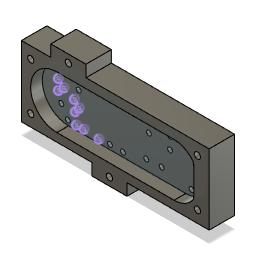
dictofun_1.3_bed_of_nails (Autodesk Fusion 360 design; units mm, degrees)
Autodesk Fusion 360 part; units mm, degrees
(part 1 of 13)
sketch "Sketch1" plane through (0, 0, 0) normal (0, 0, 1) x (1, 0, 0)
  line L0 (139.726, -70.9365) -> (139.721, -70.9397)
  line L1 (139.346, -71.4753) -> (139.289, -71.688)
  line L2 (139.439, -72.5391) -> (139.442, -72.5436)
  line L3 (139.536, -72.6768) -> (139.565, -72.7194)
  line L4 (139.906, -70.811) -> (139.906, -70.811)
  line L5 (139.439, -71.2757) -> (139.437, -71.2807)
  line L6 (139.442, -72.5436) -> (139.442, -72.5436)
  line L7 (139.846, -72.9625) -> (139.89, -73.018)
  line L8 (139.562, -71.0999) -> (139.468, -71.2339)
  line L9 (141.501, -71.0954) -> (141.345, -70.9397)
  line L10 (139.437, -72.5341) -> (139.439, -72.5391)
  line L11 (141.72, -72.3395) -> (141.777, -72.1268)
  line L12 (139.721, -70.9397) -> (139.565, -71.0954)
  line L13 (139.395, -71.3702) -> (139.346, -71.4753)
  line L14 (139.873, -80.9148) -> (139.782, -81.0293)
  line L15 (139.437, -71.2807) -> (139.437, -71.2807)
  line L16 (139.437, -71.2807) -> (139.395, -71.3702)
  line L17 (139.348, -72.3445) -> (139.437, -72.5341)
  line L18 (139.779, -72.9157) -> (139.846, -72.9625)
  line L19 (139.289, -71.688) -> (139.27, -71.9074)
  line L20 (139.565, -71.0954) -> (139.562, -71.0999)
  line L21 (139.78, -81.0344) -> (139.78, -81.0344)
  line L22 (137.742, -83.535) -> (137.082, -82.8744)
  line L23 (136.527, -82.247) -> (136.522, -82.2439)
  line L24 (139.89, -73.018) -> (139.9, -73.0658)
  line L25 (136.966, -82.6541) -> (136.891, -82.5531)
  line L26 (136.848, -82.4955) -> (136.848, -82.4955)
  line L27 (139.9, -73.0658) -> (139.9, -80.8368)
  line L28 (139.565, -72.7194) -> (139.721, -72.8751)
  line L29 (139.687, -81.2096) -> (139.627, -81.4041)
  line L30 (137.057, -82.8364) -> (137.056, -82.8368)
  line L31 (136.628, -82.3102) -> (136.527, -82.247)
  line L32 (137.788, -83.564) -> (137.742, -83.535)
  line L33 (139.437, -72.5341) -> (139.437, -72.5341)
  line L34 (136.522, -82.2439) -> (136.333, -82.1684)
  line L35 (136.969, -82.6593) -> (136.966, -82.6541)
  line L36 (139.748, -81.0945) -> (139.687, -81.2096)
  line L37 (137.056, -82.8368) -> (136.969, -82.6593)
  line L38 (137.921, -83.535) -> (137.858, -83.5691)
  line L39 (137.082, -82.8744) -> (137.057, -82.8364)
  line L40 (139.289, -72.1268) -> (139.346, -72.3395)
  line L41 (139.78, -81.0344) -> (139.748, -81.0945)
  line L42 (139.726, -72.8783) -> (139.726, -72.8783)
  line L43 (139.9, -80.8368) -> (139.88, -80.905)
  line L44 (139.609, -81.6902) -> (139.615, -81.7805)
  line L45 (139.782, -81.0293) -> (139.78, -81.0344)
  line L46 (136.891, -82.5531) -> (136.848, -82.4955)
  line L47 (136.333, -82.1684) -> (136.133, -82.1286)
  line L48 (136.848, -82.4955) -> (136.844, -82.4909)
  line L49 (137.858, -83.5691) -> (137.788, -83.564)
  line L50 (136.844, -82.4909) -> (136.695, -82.3526)
  line L51 (139.627, -81.4041) -> (139.603, -81.6065)
  line L52 (139.599, -81.8497) -> (139.578, -81.8778)
  line L53 (136.105, -81.7081) -> (136.105, -81.7081)
  line L54 (136.128, -82.1286) -> (136.122, -82.128)
  line L55 (136.108, -81.6604) -> (136.11, -81.6482)
  line L56 (136.105, -81.7081) -> (136.107, -81.7004)
  line L57 (139.721, -72.8751) -> (139.726, -72.8783)
  line L58 (139.726, -72.8783) -> (139.779, -72.9157)
  line L59 (139.603, -81.6065) -> (139.609, -81.6902)
  line L60 (139.27, -71.9074) -> (139.289, -72.1268)
  line L61 (139.88, -80.905) -> (139.873, -80.9148)
  line L62 (136.133, -82.1286) -> (136.128, -82.1286)
  line L63 (139.562, -71.0999) -> (139.562, -71.0999)
  line L64 (139.442, -72.5436) -> (139.536, -72.6768)
  line L65 (139.578, -81.8778) -> (137.921, -83.535)
  line L66 (136.527, -82.247) -> (136.527, -82.247)
  line L67 (139.346, -72.3395) -> (139.348, -72.3445)
  line L68 (136.695, -82.3526) -> (136.628, -82.3102)
  line L69 (136.122, -82.128) -> (136.122, -82.1254)
  line L70 (139.468, -71.2339) -> (139.439, -71.2757)
  line L71 (139.615, -81.7805) -> (139.599, -81.8497)
  line L72 (136.127, -72.9976) -> (136.161, -72.9625)
  line L73 (136.046, -81.8942) -> (136.067, -81.8554)
  line L74 (136.065, -82.1077) -> (136.019, -82.0534)
  line L75 (136.083, -81.8058) -> (136.087, -81.7985)
  line L76 (136.023, -81.9456) -> (136.023, -81.9454)
  line L77 (136.088, -81.7907) -> (136.094, -81.7548)
  line L78 (136.096, -81.7432) -> (136.105, -81.7081)
  line L79 (136.088, -81.7907) -> (136.088, -81.7907)
  line L80 (136.069, -81.8477) -> (136.069, -81.8477)
  line L81 (136.161, -72.9625) -> (136.228, -72.9157)
  line L82 (136.112, -81.6404) -> (136.107, -81.5964)
  line L83 (136.564, -72.5436) -> (136.564, -72.5436)
  line L84 (136.087, -81.7985) -> (136.088, -81.7907)
  line L85 (136.01, -81.983) -> (136.023, -81.9456)
  line L86 (136.57, -72.5341) -> (136.658, -72.3445)
  line L87 (136.718, -72.1268) -> (136.737, -71.9074)
  line L88 (136.228, -72.9157) -> (136.281, -72.8783)
  line L89 (136.107, -73.0658) -> (136.127, -72.9976)
  line L90 (136.107, -81.5845) -> (136.107, -73.0658)
  line L91 (136.11, -81.6482) -> (136.112, -81.6404)
  line L92 (136.072, -81.8358) -> (136.079, -81.8171)
  line L93 (136.122, -82.1254) -> (136.065, -82.1077)
  line L94 (136.067, -81.8554) -> (136.069, -81.8477)
  line L95 (136.079, -81.8171) -> (136.083, -81.8058)
  line L96 (136.019, -82.0534) -> (136.01, -81.983)
  line L97 (136.094, -81.7548) -> (136.096, -81.7432)
  line L98 (136.107, -81.7004) -> (136.107, -81.6801)
  line L99 (136.107, -81.6801) -> (136.108, -81.6604)
  line L100 (136.023, -81.9454) -> (136.023, -81.9454)
  line L101 (136.069, -81.8477) -> (136.072, -81.8358)
  line L102 (136.57, -72.5341) -> (136.57, -72.5341)
  line L103 (136.281, -72.8783) -> (136.281, -72.8783)
  line L104 (136.281, -72.8783) -> (136.285, -72.8751)
  line L105 (136.023, -81.9454) -> (136.041, -81.9048)
  line L106 (136.285, -70.9397) -> (136.105, -70.8133)
  line L107 (136.285, -72.8751) -> (136.441, -72.7194)
  line L108 (136.567, -72.5391) -> (136.57, -72.5341)
  line L109 (136.107, -81.5964) -> (136.107, -81.5845)
  line L110 (136.105, -70.8133) -> (135.906, -70.7203)
  line L111 (135.906, -70.7203) -> (135.693, -70.6633)
  line L112 (135.468, -70.6446) -> (135.462, -70.6446)
  line L113 (136.041, -81.9048) -> (136.046, -81.8942)
  line L114 (152.42, -70.6251) -> (152.301, -70.4493)
  line L115 (135.473, -70.6441) -> (135.468, -70.6446)
  line L116 (136.718, -71.688) -> (136.661, -71.4753)
  line L117 (136.471, -72.6768) -> (136.564, -72.5436)
  line L118 (152.642, -69.2633) -> (152.654, -69.3169)
  line L119 (136.661, -72.3395) -> (136.718, -72.1268)
  line L120 (136.441, -72.7194) -> (136.471, -72.6768)
  line L121 (151.93, -70.1136) -> (151.926, -70.1105)
  line L122 (152.129, -70.2665) -> (152.125, -70.2628)
  line L123 (135.462, -70.6446) -> (135.462, -70.6434)
  line L124 (136.564, -72.5436) -> (136.567, -72.5391)
  line L125 (136.444, -71.0999) -> (136.441, -71.0954)
  line L126 (152.442, -70.6493) -> (152.42, -70.6251)
  line L127 (152.301, -70.4493) -> (152.298, -70.4451)
  line L128 (152.506, -70.679) -> (152.442, -70.6493)
  line L129 (152.121, -70.2598) -> (151.93, -70.1136)
  line L130 (135.351, -69.3736) -> (135.405, -69.3271)
  line L131 (152.527, -69.1905) -> (152.595, -69.21)
  line L132 (136.444, -71.0999) -> (136.444, -71.0999)
  line L133 (136.567, -71.2757) -> (136.538, -71.2339)
  line L134 (135.693, -70.6633) -> (135.473, -70.6441)
  line L135 (136.737, -71.9074) -> (136.718, -71.688)
  line L136 (136.661, -71.4753) -> (136.612, -71.3702)
  line L137 (136.538, -71.2339) -> (136.444, -71.0999)
  line L138 (136.57, -71.2807) -> (136.567, -71.2757)
  line L139 (136.612, -71.3702) -> (136.57, -71.2807)
  line L140 (135.331, -69.4417) -> (135.351, -69.3736)
  line L141 (136.441, -71.0954) -> (136.285, -70.9397)
  line L142 (135.456, -69.3157) -> (152.527, -69.1905)
  line L143 (151.7, -69.9904) -> (151.473, -69.912)
  line L144 (136.658, -72.3445) -> (136.661, -72.3395)
  line L145 (152.63, -70.6227) -> (152.576, -70.6691)
  line L146 (135.462, -70.6434) -> (135.399, -70.6306)
  line L147 (136.57, -71.2807) -> (136.57, -71.2807)
  line L148 (135.405, -69.3271) -> (135.456, -69.3157)
  line L149 (152.595, -69.21) -> (152.642, -69.2633)
  line L150 (151.93, -70.1136) -> (151.93, -70.1136)
  line L151 (135.348, -70.5812) -> (135.331, -70.519)
  line L152 (141.63, -71.2807) -> (141.629, -71.2807)
  line L153 (141.504, -71.0999) -> (141.501, -71.0954)
  line L154 (141.668, -81.0591) -> (141.665, -81.0539)
  line L155 (141.805, -81.8497) -> (141.828, -81.6939)
  line L156 (141.225, -80.6462) -> (141.178, -80.5929)
  line L157 (141.811, -81.4327) -> (141.755, -81.2366)
  line L158 (141.777, -72.1268) -> (141.796, -71.9074)
  line L159 (141.629, -71.2807) -> (141.627, -71.2757)
  line L160 (141.72, -71.4753) -> (141.671, -71.3702)
  line L161 (139.901, -70.8133) -> (139.897, -70.8165)
  line L162 (139.897, -70.8165) -> (139.726, -70.9365)
  line L163 (140.533, -70.6441) -> (140.314, -70.6633)
  line L164 (139.897, -70.8165) -> (139.897, -70.8165)
  line L165 (141.718, -72.3445) -> (141.72, -72.3395)
  line L166 (141.627, -71.2757) -> (141.598, -71.2339)
  line L167 (141.598, -71.2339) -> (141.504, -71.0999)
  line L168 (141.345, -70.9397) -> (141.165, -70.8133)
  line L169 (141.187, -72.9976) -> (141.22, -72.9625)
  line L170 (141.63, -72.5341) -> (141.718, -72.3445)
  line L171 (140.965, -70.7203) -> (140.752, -70.6633)
  line L172 (141.167, -80.5396) -> (141.167, -73.0658)
  line L173 (141.884, -81.999) -> (141.827, -81.9564)
  line L174 (141.671, -71.3702) -> (141.63, -71.2807)
  line L175 (141.777, -71.688) -> (141.72, -71.4753)
  line L176 (140.101, -70.7203) -> (140.008, -70.7638)
  line L177 (141.796, -71.9074) -> (141.777, -71.688)
  line L178 (140.314, -70.6633) -> (140.101, -70.7203)
  line L179 (140.752, -70.6633) -> (140.533, -70.6441)
  line L180 (140.008, -70.7638) -> (139.906, -70.811)
  line L181 (139.906, -70.811) -> (139.901, -70.8133)
  line L182 (139.726, -70.9365) -> (139.726, -70.9365)
  line L183 (141.629, -72.5341) -> (141.63, -72.5341)
  line L184 (141.504, -71.0999) -> (141.504, -71.0999)
  line L185 (141.165, -70.8133) -> (140.965, -70.7203)
  line L186 (151.238, -96.6842) -> (151.233, -96.6793)
  line L187 (151.626, -97.4609) -> (151.621, -97.4545)
  line L188 (151.682, -97.5383) -> (151.66, -97.5002)
  line L189 (150.656, -96.4497) -> (150.588, -96.4297)
  line L190 (151.073, -96.5644) -> (150.91, -96.4921)
  line L191 (151.697, -97.5595) -> (151.689, -97.5482)
  line L192 (150.724, -96.4511) -> (150.717, -96.4497)
  line L193 (151.079, -96.5671) -> (151.073, -96.5644)
  line L194 (150.53, -96.3237) -> (150.53, -96.3063)
  line L195 (150.542, -96.376) -> (150.53, -96.3237)
  line L196 (150.838, -95.573) -> (150.818, -95.3831)
  line L197 (150.659, -96.1149) -> (150.664, -96.11)
  line L198 (151.646, -97.4859) -> (151.633, -97.4709)
  line L199 (151.073, -96.5644) -> (151.073, -96.5644)
  line L200 (151.533, -97.3335) -> (151.516, -97.1748)
  line L201 (151.516, -97.1748) -> (151.516, -97.1748)
  line L202 (150.717, -96.4497) -> (150.656, -96.4497)
  line L203 (151.689, -97.5482) -> (151.682, -97.5383)
  line L204 (150.756, -95.9503) -> (150.759, -95.9446)
  line L205 (150.759, -95.9446) -> (150.818, -95.763)
  line L206 (150.818, -95.763) -> (150.824, -95.7052)
  line L207 (151.516, -97.1683) -> (151.457, -96.9866)
  line L208 (150.53, -96.3063) -> (150.551, -96.2382)
  line L209 (151.238, -96.6842) -> (151.238, -96.6842)
  line L210 (151.731, -97.6206) -> (151.722, -97.6028)
  line L211 (151.578, -97.4183) -> (151.569, -97.4094)
  line L212 (151.621, -97.4545) -> (151.587, -97.4263)
  line L213 (151.516, -97.1748) -> (151.516, -97.1683)
  line L214 (151.535, -97.3471) -> (151.533, -97.3335)
  line L215 (151.233, -96.6793) -> (151.079, -96.5671)
  line L216 (151.66, -97.5002) -> (151.646, -97.4859)
  line L217 (151.569, -97.4094) -> (151.535, -97.3471)
  line L218 (151.457, -96.9866) -> (151.361, -96.8213)
  line L219 (150.54, -94.8991) -> (150.54, -94.8991)
  line L220 (150.818, -95.3831) -> (150.759, -95.2015)
  line L221 (150.659, -96.1149) -> (150.659, -96.1149)
  line L222 (150.91, -96.4921) -> (150.904, -96.4894)
  line L223 (150.588, -96.4297) -> (150.542, -96.376)
  line L224 (150.722, -96.009) -> (150.756, -95.9503)
  line L225 (150.664, -95.0361) -> (150.594, -94.9585)
  line L226 (150.759, -95.2015) -> (150.664, -95.0361)
  line L227 (150.91, -96.4921) -> (150.91, -96.4921)
  line L228 (150.904, -96.4894) -> (150.811, -96.4696)
  line L229 (150.563, -96.222) -> (150.568, -96.2167)
  line L230 (150.724, -96.4511) -> (150.724, -96.4511)
  line L231 (150.756, -95.9503) -> (150.756, -95.9503)
  line L232 (150.837, -95.5796) -> (150.838, -95.573)
  line L233 (150.811, -96.4696) -> (150.724, -96.4511)
  line L234 (150.551, -96.2382) -> (150.563, -96.222)
  line L235 (150.664, -96.11) -> (150.722, -96.009)
  line L236 (150.594, -94.9585) -> (150.54, -94.8991)
  line L237 (150.588, -96.194) -> (150.659, -96.1149)
  line L238 (149.474, -94.7792) -> (149.474, -94.7792)
  line L239 (149.736, -94.6844) -> (149.642, -94.7042)
  line L240 (149.309, -94.8991) -> (149.309, -94.8991)
  line L241 (150.114, -94.6844) -> (150.027, -94.6659)
  line L242 (149.256, -94.9585) -> (149.186, -95.0361)
  line L243 (150.027, -94.6659) -> (150.02, -94.6645)
  line L244 (149.313, -94.8942) -> (149.309, -94.8991)
  line L245 (150.387, -94.7858) -> (150.381, -94.7819)
  line L246 (150.536, -94.8942) -> (150.402, -94.7967)
  line L247 (150.824, -95.7052) -> (150.837, -95.5796)
  line L248 (149.823, -94.6659) -> (149.823, -94.6659)
  line L249 (149.309, -94.8991) -> (149.256, -94.9585)
  line L250 (150.568, -96.2167) -> (150.588, -96.194)
  line L251 (149.829, -94.6645) -> (149.823, -94.6659)
  line L252 (149.823, -94.6659) -> (149.736, -94.6844)
  line L253 (150.375, -94.7792) -> (150.213, -94.7069)
  line L254 (150.027, -94.6659) -> (150.027, -94.6659)
  line L255 (149.468, -94.7819) -> (149.463, -94.7858)
  line L256 (149.463, -94.7858) -> (149.463, -94.7858)
  line L257 (150.375, -94.7792) -> (150.375, -94.7792)
  line L258 (149.642, -94.7042) -> (149.636, -94.7069)
  line L259 (149.636, -94.7069) -> (149.474, -94.7792)
  line L260 (150.213, -94.7069) -> (150.207, -94.7042)
  line L261 (150.02, -94.6645) -> (149.829, -94.6645)
  line L262 (150.54, -94.8991) -> (150.536, -94.8942)
  line L263 (149.636, -94.7069) -> (149.636, -94.7069)
  line L264 (151.744, -97.6456) -> (151.744, -97.6456)
  line L265 (151.722, -97.6028) -> (151.718, -97.5914)
  line L266 (151.718, -97.5914) -> (151.715, -97.584)
  line L267 (151.361, -96.8213) -> (151.354, -96.8129)
  line L268 (151.633, -97.4709) -> (151.626, -97.4609)
  line L269 (151.587, -97.4263) -> (151.578, -97.4183)
  line L270 (151.715, -97.584) -> (151.697, -97.5595)
  line L271 (151.354, -96.8129) -> (151.238, -96.6842)
  line L272 (109.339, -72.2892) -> (109.319, -72.2735)
  line L273 (109.218, -72.1062) -> (109.229, -72.0294)
  line L274 (110.091, -71.3039) -> (110.048, -71.2465)
  line L275 (110.253, -71.0302) -> (110.273, -71.0459)
  line L276 (110.088, -70.9143) -> (110.093, -70.9159)
  line L277 (110.427, -70.208) -> (110.43, -70.2113)
  line L278 (110.085, -70.9108) -> (110.088, -70.9143)
  line L279 (110.365, -72.141) -> (110.352, -72.1584)
  line L280 (110.093, -72.4036) -> (110.088, -72.4052)
  line L281 (110.236, -72.3083) -> (110.093, -72.4036)
  line L282 (110.01, -72.4288) -> (109.581, -72.4288)
  line L283 (109.791, -71.1895) -> (109.787, -71.1904)
  line L284 (109.277, -71.9683) -> (109.349, -71.9394)
  line L285 (110.365, -71.1785) -> (110.436, -71.369)
  line L286 (110.273, -72.2735) -> (110.253, -72.2892)
  line L287 (109.718, -71.1675) -> (109.713, -71.1661)
  line L288 (109.319, -72.2735) -> (109.247, -72.1783)
  line L289 (109.229, -72.0294) -> (109.277, -71.9683)
  line L290 (110.446, -71.4216) -> (110.446, -71.8978)
  line L291 (110.064, -70.9052) -> (110.085, -70.9108)
  line L292 (110.085, -72.4087) -> (110.052, -72.4175)
  line L293 (109.539, -72.4175) -> (109.506, -72.4087)
  line L294 (103.221, -70.8155) -> (103.296, -70.7954)
  line L295 (109.787, -71.1904) -> (109.754, -71.1795)
  line L296 (110.052, -72.4175) -> (110.02, -72.4284)
  line L297 (110.435, -70.3203) -> (110.426, -70.3538)
  line L298 (110.015, -72.4275) -> (110.01, -72.4288)
  line L299 (110.439, -71.3957) -> (110.446, -71.4216)
  line L300 (109.498, -72.4036) -> (109.355, -72.3083)
  line L301 (109.247, -72.1783) -> (109.218, -72.1062)
  line L302 (110.088, -72.4052) -> (110.085, -72.4087)
  line L303 (110.344, -72.1783) -> (110.273, -72.2735)
  line L304 (110.446, -71.8978) -> (110.439, -71.9238)
  line L305 (110.236, -71.0111) -> (110.253, -71.0302)
  line L306 (110.344, -71.1411) -> (110.352, -71.161)
  line L307 (110.253, -72.2892) -> (110.236, -72.3083)
  line L308 (110.146, -71.8706) -> (110.146, -71.4488)
  line L309 (110.146, -71.4488) -> (110.091, -71.3039)
  line L310 (109.796, -71.1907) -> (109.791, -71.1895)
  line L311 (109.349, -71.9394) -> (109.426, -71.9503)
  line L312 (109.754, -71.1795) -> (109.721, -71.1706)
  line L313 (109.506, -72.4087) -> (109.503, -72.4052)
  line L314 (110.048, -71.2465) -> (109.965, -71.1907)
  line L315 (110.445, -70.2873) -> (110.435, -70.3203)
  line L316 (110.421, -70.3611) -> (110.064, -70.9052)
  line L317 (110.273, -71.0459) -> (110.344, -71.1411)
  line L318 (109.721, -71.1706) -> (109.718, -71.1675)
  line L319 (110.02, -72.4284) -> (110.015, -72.4275)
  line L320 (110.422, -70.3569) -> (110.421, -70.3611)
  line L321 (110.436, -71.9505) -> (110.365, -72.141)
  line L322 (110.352, -71.161) -> (110.365, -71.1785)
  line L323 (109.355, -72.3083) -> (109.339, -72.2892)
  line L324 (110.352, -72.1584) -> (110.344, -72.1783)
  line L325 (109.965, -71.1907) -> (109.796, -71.1907)
  line L326 (109.543, -72.073) -> (109.627, -72.1288)
  line L327 (110.436, -71.369) -> (110.439, -71.3957)
  line L328 (109.503, -72.4052) -> (109.498, -72.4036)
  line L329 (110.093, -70.9159) -> (110.236, -71.0111)
  line L330 (109.581, -72.4288) -> (109.577, -72.4275)
  line L331 (109.577, -72.4275) -> (109.572, -72.4284)
  line L332 (109.965, -72.1288) -> (110.048, -72.073)
  line L333 (110.439, -71.9238) -> (110.436, -71.9505)
  line L334 (110.048, -72.073) -> (110.091, -72.0155)
  line L335 (109.487, -71.9983) -> (109.543, -72.073)
  line L336 (102.005, -72.4275) -> (102, -72.4284)
  line L337 (101.946, -71.0954) -> (101.946, -71.9658)
  line L338 (101.727, -72.2362) -> (101.655, -72.0457)
  line L339 (102.303, -72.2788) -> (102.283, -72.3538)
  line L340 (102.01, -72.4288) -> (102.005, -72.4275)
  line L341 (109.627, -72.1288) -> (109.965, -72.1288)
  line L342 (109.646, -71.0407) -> (109.647, -71.0364)
  line L343 (109.69, -71.1402) -> (109.666, -71.1157)
  line L344 (109.367, -70.4288) -> (109.292, -70.4087)
  line L345 (109.655, -71.0742) -> (109.646, -71.0407)
  line L346 (109.657, -70.9992) -> (109.666, -70.9657)
  line L347 (109.237, -70.2038) -> (109.292, -70.1489)
  line L348 (109.367, -70.1288) -> (110.296, -70.1288)
  line L349 (109.572, -72.4284) -> (109.539, -72.4175)
  line L350 (110.091, -72.0155) -> (110.146, -71.8706)
  line L351 (109.713, -71.1661) -> (109.69, -71.1402)
  line L352 (109.646, -71.0321) -> (109.657, -70.9992)
  line L353 (110.296, -70.1288) -> (110.3, -70.1299)
  line L354 (109.662, -71.1081) -> (109.655, -71.0742)
  line L355 (109.426, -71.9503) -> (109.487, -71.9983)
  line L356 (101.926, -70.2038) -> (101.946, -70.2788)
  line L357 (109.67, -70.9584) -> (110.018, -70.4288)
  line L358 (110.018, -70.4288) -> (109.367, -70.4288)
  line L359 (109.647, -71.0364) -> (109.646, -71.0321)
  line L360 (109.669, -70.9625) -> (109.67, -70.9584)
  line L361 (102.283, -70.8704) -> (102.303, -70.9454)
  line L362 (109.666, -70.9657) -> (109.669, -70.9625)
  line L363 (102.303, -70.9454) -> (102.283, -71.0204)
  line L364 (109.665, -71.1114) -> (109.662, -71.1081)
  line L365 (102.283, -71.0204) -> (102.228, -71.0753)
  line L366 (101.927, -72.4036) -> (101.784, -72.3083)
  line L367 (109.217, -70.2788) -> (109.237, -70.2038)
  line L368 (109.666, -71.1157) -> (109.665, -71.1114)
  line L369 (101.871, -70.1489) -> (101.926, -70.2038)
  line L370 (101.946, -70.7954) -> (102.153, -70.7954)
  line L371 (109.237, -70.3538) -> (109.217, -70.2788)
  line L372 (109.292, -70.4087) -> (109.237, -70.3538)
  line L373 (101.946, -70.2788) -> (101.946, -70.7954)
  line L374 (102.153, -70.7954) -> (102.228, -70.8155)
  line L375 (109.292, -70.1489) -> (109.367, -70.1288)
  line L376 (102.228, -70.8155) -> (102.283, -70.8704)
  line L377 (102.228, -71.0753) -> (102.153, -71.0954)
  line L378 (101.796, -70.1288) -> (101.871, -70.1489)
  line L379 (101.451, -70.8704) -> (101.506, -70.8155)
  line L380 (101.646, -70.2788) -> (101.666, -70.2038)
  line L381 (101.451, -71.0204) -> (101.431, -70.9454)
  line L382 (91.0684, -70.2038) -> (91.0885, -70.2788)
  line L383 (102.228, -72.4087) -> (102.153, -72.4288)
  line L384 (101.991, -72.0856) -> (102.055, -72.1288)
  line L385 (101.646, -71.993) -> (101.646, -71.0954)
  line L386 (91.2957, -72.1288) -> (91.3707, -72.1489)
  line L387 (91.3707, -70.8155) -> (91.4256, -70.8704)
  line L388 (101.753, -72.2737) -> (101.733, -72.25)
  line L389 (101.655, -72.0457) -> (101.653, -72.019)
  line L390 (101.731, -72.2425) -> (101.727, -72.2362)
  line L391 (101.931, -72.4052) -> (101.927, -72.4036)
  line L392 (101.772, -72.2994) -> (101.753, -72.2737)
  line L393 (101.784, -72.3083) -> (101.779, -72.3025)
  line L394 (102.153, -72.4288) -> (102.01, -72.4288)
  line L395 (101.653, -72.019) -> (101.646, -71.993)
  line L396 (101.646, -71.0954) -> (101.581, -71.0954)
  line L397 (101.581, -71.0954) -> (101.506, -71.0753)
  line L398 (91.4256, -72.2038) -> (91.4457, -72.2788)
  line L399 (101.733, -72.25) -> (101.731, -72.2425)
  line L400 (101.506, -71.0753) -> (101.451, -71.0204)
  line L401 (101.506, -70.8155) -> (101.581, -70.7954)
  line L402 (91.4256, -72.3538) -> (91.3707, -72.4087)
  line L403 (91.3707, -72.4087) -> (91.2957, -72.4288)
  line L404 (91.0135, -70.1489) -> (91.0684, -70.2038)
  line L405 (102.153, -72.1288) -> (102.228, -72.1489)
  line L406 (101.779, -72.3025) -> (101.772, -72.2994)
  line L407 (102, -72.4284) -> (101.968, -72.4175)
  line L408 (91.4457, -72.2788) -> (91.4256, -72.3538)
  line L409 (101.935, -72.4087) -> (101.931, -72.4052)
  line L410 (102.228, -72.1489) -> (102.283, -72.2038)
  line L411 (91.2957, -70.7954) -> (91.3707, -70.8155)
  line L412 (102.055, -72.1288) -> (102.153, -72.1288)
  line L413 (101.666, -70.2038) -> (101.721, -70.1489)
  line L414 (102.283, -72.2038) -> (102.303, -72.2788)
  line L415 (101.431, -70.9454) -> (101.451, -70.8704)
  line L416 (101.646, -70.7954) -> (101.646, -70.2788)
  line L417 (101.946, -71.9658) -> (101.991, -72.0856)
  line L418 (102.283, -72.3538) -> (102.228, -72.4087)
  line L419 (91.2957, -72.4288) -> (91.1528, -72.4288)
  line L420 (102.153, -71.0954) -> (101.946, -71.0954)
  line L421 (101.968, -72.4175) -> (101.935, -72.4087)
  line L422 (90.9385, -70.1288) -> (91.0135, -70.1489)
  line L423 (90.7243, -71.0954) -> (90.6493, -71.0753)
  line L424 (90.6493, -70.8155) -> (90.7243, -70.7954)
  line L425 (90.7981, -72.0457) -> (90.7955, -72.019)
  line L426 (90.8635, -70.1489) -> (90.9385, -70.1288)
  line L427 (101.721, -70.1489) -> (101.796, -70.1288)
  line L428 (91.148, -72.4275) -> (91.1432, -72.4284)
  line L429 (90.7885, -70.7954) -> (90.7885, -70.2788)
  line L430 (90.7885, -70.2788) -> (90.8086, -70.2038)
  line L431 (91.0743, -72.4052) -> (91.0696, -72.4036)
  line L432 (91.0885, -71.0954) -> (91.0885, -71.9658)
  line L433 (90.8963, -72.2737) -> (90.8755, -72.25)
  line L434 (91.2957, -71.0954) -> (91.0885, -71.0954)
  line L435 (90.9147, -72.2994) -> (90.8963, -72.2737)
  line L436 (91.1108, -72.4175) -> (91.0778, -72.4087)
  line L437 (99.7372, -72.3538) -> (99.7171, -72.2788)
  line L438 (88.8635, -70.8155) -> (88.9385, -70.7954)
  line L439 (99.997, -70.8704) -> (100.017, -70.9454)
  line L440 (91.1432, -72.4284) -> (91.1108, -72.4175)
  line L441 (88.8086, -70.8704) -> (88.8635, -70.8155)
  line L442 (99.7372, -70.8704) -> (99.7921, -70.8155)
  line L443 (100.017, -70.9454) -> (100.017, -72.2788)
  line L444 (90.7243, -70.7954) -> (90.7885, -70.7954)
  line L445 (91.4256, -71.0204) -> (91.3707, -71.0753)
  line L446 (90.5944, -70.8704) -> (90.6493, -70.8155)
  line L447 (90.5944, -71.0204) -> (90.5743, -70.9454)
  line L448 (91.0885, -70.2788) -> (91.0885, -70.7954)
  line L449 (91.3707, -71.0753) -> (91.2957, -71.0954)
  line L450 (90.9268, -72.3083) -> (90.9217, -72.3025)
  line L451 (91.1334, -72.0856) -> (91.1982, -72.1288)
  line L452 (90.9217, -72.3025) -> (90.9147, -72.2994)
  line L453 (90.5743, -70.9454) -> (90.5944, -70.8704)
  line L454 (89.0684, -70.8704) -> (89.0885, -70.9454)
  line L455 (90.7955, -72.019) -> (90.7885, -71.993)
  line L456 (91.0778, -72.4087) -> (91.0743, -72.4052)
  line L457 (90.8695, -72.2362) -> (90.7981, -72.0457)
  line L458 (99.2957, -70.4288) -> (98.7314, -70.4288)
  line L459 (99.7921, -72.4087) -> (99.7372, -72.3538)
  line L460 (90.7885, -71.0954) -> (90.7243, -71.0954)
  line L461 (91.1528, -72.4288) -> (91.148, -72.4275)
  line L462 (99.3707, -70.1489) -> (99.4256, -70.2038)
  line L463 (99.9421, -70.8155) -> (99.997, -70.8704)
  line L464 (91.4457, -70.9454) -> (91.4256, -71.0204)
  line L465 (91.4256, -70.8704) -> (91.4457, -70.9454)
  line L466 (90.7885, -71.993) -> (90.7885, -71.0954)
  line L467 (90.874, -72.2425) -> (90.8695, -72.2362)
  line L468 (90.8086, -70.2038) -> (90.8635, -70.1489)
  line L469 (91.3707, -72.1489) -> (91.4256, -72.2038)
  line L470 (91.0885, -71.9658) -> (91.1334, -72.0856)
  line L471 (99.8671, -72.4288) -> (99.7921, -72.4087)
  line L472 (99.7171, -72.2788) -> (99.7171, -70.9454)
  line L473 (88.8086, -72.3538) -> (88.7885, -72.2788)
  line L474 (99.7921, -70.8155) -> (99.8671, -70.7954)
  line L475 (91.1982, -72.1288) -> (91.2957, -72.1288)
  line L476 (91.0696, -72.4036) -> (90.9268, -72.3083)
  line L477 (88.9385, -72.4288) -> (88.8635, -72.4087)
  line L478 (99.9421, -72.4087) -> (99.8671, -72.4288)
  line L479 (91.0885, -70.7954) -> (91.2957, -70.7954)
  line L480 (89.0135, -70.8155) -> (89.0684, -70.8704)
  line L481 (89.0885, -72.2788) -> (89.0684, -72.3538)
  line L482 (101.581, -70.7954) -> (101.646, -70.7954)
  line L483 (90.6493, -71.0753) -> (90.5944, -71.0204)
  line L484 (90.8755, -72.25) -> (90.874, -72.2425)
  line L485 (88.8635, -72.4087) -> (88.8086, -72.3538)
  line L486 (95.8801, -72.3538) -> (95.86, -72.2788)
  line L487 (95.2921, -72.4087) -> (95.2372, -72.3538)
  line L488 (99.3707, -70.4087) -> (99.2957, -70.4288)
  line L489 (95.4421, -70.8155) -> (95.4676, -70.841)
  line L490 (99.997, -72.3538) -> (99.9421, -72.4087)
  line L491 (95.8005, -70.7967) -> (95.8053, -70.7957)
  line L492 (95.935, -72.4087) -> (95.8801, -72.3538)
  line L493 (95.5171, -72.2788) -> (95.497, -72.3538)
  line L494 (95.8377, -70.8067) -> (95.8707, -70.8155)
  line L495 (99.2113, -71.3061) -> (99.1564, -71.361)
  line L496 (98.7314, -72.2788) -> (98.7113, -72.3538)
  line L497 (99.0814, -71.3811) -> (98.7314, -71.3811)
  line L498 (99.4256, -70.3538) -> (99.3707, -70.4087)
  line L499 (88.9385, -70.7954) -> (89.0135, -70.8155)
  line L500 (98.5064, -70.1489) -> (98.5814, -70.1288)
  line L501 (99.1564, -71.1012) -> (99.2113, -71.1561)
  line L502 (96.0268, -70.9216) -> (96.0338, -70.9248)
  line L503 (99.2314, -71.2311) -> (99.2113, -71.3061)
  line L504 (89.0684, -72.3538) -> (89.0135, -72.4087)
  line L505 (96.0522, -70.9505) -> (96.073, -70.9742)
  line L506 (99.8671, -70.7954) -> (99.9421, -70.8155)
  line L507 (88.7885, -72.2788) -> (88.7885, -70.9454)
  line L508 (95.8053, -70.7957) -> (95.8377, -70.8067)
  line L509 (99.1564, -71.361) -> (99.0814, -71.3811)
  line L510 (100.017, -72.2788) -> (99.997, -72.3538)
  line L511 (98.4314, -70.2788) -> (98.4515, -70.2038)
  line L512 (96.0217, -70.9159) -> (96.0268, -70.9216)
  line L513 (95.8789, -70.8206) -> (96.0217, -70.9159)
  line L514 (98.7113, -72.3538) -> (98.6564, -72.4087)
  line L515 (98.5064, -72.4087) -> (98.4515, -72.3538)
  line L516 (99.4457, -70.2788) -> (99.4256, -70.3538)
  line L517 (98.5814, -72.4288) -> (98.5064, -72.4087)
  line L518 (98.4314, -72.2788) -> (98.4314, -70.2788)
  line L519 (95.5171, -71.1859) -> (95.5171, -72.2788)
  line L520 (95.4421, -72.4087) -> (95.3671, -72.4288)
  line L521 (95.2171, -72.2788) -> (95.2171, -70.9454)
  line L522 (99.7171, -70.9454) -> (99.7372, -70.8704)
  line L523 (99.4256, -70.2038) -> (99.4457, -70.2788)
  line L524 (96.01, -72.4288) -> (95.935, -72.4087)
  line L525 (96.0338, -70.9248) -> (96.0522, -70.9505)
  line L526 (95.5431, -71.1512) -> (95.5171, -71.1859)
  line L527 (95.2921, -70.8155) -> (95.3671, -70.7954)
  line L528 (95.6268, -71.0954) -> (95.5431, -71.1512)
  line L529 (98.4515, -72.3538) -> (98.4314, -72.2788)
  line L530 (96.1504, -71.1785) -> (96.153, -71.2052)
  line L531 (98.7314, -70.4288) -> (98.7314, -71.0811)
  line L532 (98.7314, -71.0811) -> (99.0814, -71.0811)
  line L533 (98.5814, -70.1288) -> (99.2957, -70.1288)
  line L534 (89.0135, -72.4087) -> (88.9385, -72.4288)
  line L535 (99.2957, -70.1288) -> (99.3707, -70.1489)
  line L536 (98.4515, -70.2038) -> (98.5064, -70.1489)
  line L537 (99.2113, -71.1561) -> (99.2314, -71.2311)
  line L538 (88.7885, -70.9454) -> (88.8086, -70.8704)
  line L539 (89.0885, -70.9454) -> (89.0885, -72.2788)
  line L540 (99.0814, -71.0811) -> (99.1564, -71.1012)
  line L541 (96.1399, -72.3538) -> (96.085, -72.4087)
  line L542 (96.085, -72.4087) -> (96.01, -72.4288)
  line L543 (98.7314, -71.3811) -> (98.7314, -72.2788)
  line L544 (95.8707, -70.8155) -> (95.8742, -70.819)
  line L545 (95.8742, -70.819) -> (95.8789, -70.8206)
  line L546 (95.3671, -70.7954) -> (95.4421, -70.8155)
  line L547 (96.153, -71.2052) -> (96.16, -71.2311)
  line L548 (98.6564, -72.4087) -> (98.5814, -72.4288)
  line L549 (95.4676, -70.841) -> (95.4982, -70.8206)
  line L550 (95.7503, -71.0954) -> (95.6268, -71.0954)
  line L551 (95.8151, -71.1386) -> (95.7503, -71.0954)
  line L552 (89.9125, -72.1288) -> (90.1074, -72.1288)
  line L553 (95.5766, -70.7967) -> (95.5814, -70.7954)
  line L554 (95.497, -72.3538) -> (95.4421, -72.4087)
  line L555 (95.86, -72.2788) -> (95.86, -71.2583)
  line L556 (95.4982, -70.8206) -> (95.5029, -70.819)
  line L557 (89.7314, -71.8706) -> (89.7857, -72.0155)
  line L558 (90.236, -70.8206) -> (90.3789, -70.9159)
  line L559 (95.5717, -70.7957) -> (95.5766, -70.7967)
  line L560 (95.5814, -70.7954) -> (95.7957, -70.7954)
  line L561 (95.7957, -70.7954) -> (95.8005, -70.7967)
  line L562 (89.8288, -71.1512) -> (89.7857, -71.2087)
  line L563 (95.86, -71.2583) -> (95.8151, -71.1386)
  line L564 (89.8288, -72.073) -> (89.9125, -72.1288)
  line L565 (90.1948, -70.8067) -> (90.2278, -70.8155)
  line L566 (90.2313, -70.819) -> (90.236, -70.8206)
  line L567 (95.2372, -70.8704) -> (95.2921, -70.8155)
  line L568 (96.0745, -70.9817) -> (96.079, -70.988)
  line L569 (95.3671, -72.4288) -> (95.2921, -72.4087)
  line L570 (95.2372, -72.3538) -> (95.2171, -72.2788)
  line L571 (89.7857, -72.0155) -> (89.8288, -72.073)
  line L572 (96.079, -70.988) -> (96.1504, -71.1785)
  line L573 (90.2125, -72.0587) -> (90.286, -72.0338)
  line L574 (90.3622, -71.1751) -> (90.286, -71.1904)
  line L575 (90.2125, -71.1655) -> (90.1074, -71.0954)
  line L576 (89.7857, -71.2087) -> (89.7314, -71.3536)
  line L577 (89.7314, -71.3536) -> (89.7314, -71.8706)
  line L578 (90.4205, -71.1239) -> (90.3622, -71.1751)
  line L579 (90.1576, -70.7967) -> (90.1625, -70.7957)
  line L580 (90.4301, -70.9742) -> (90.4454, -71.0503)
  line L581 (95.5394, -70.8067) -> (95.5717, -70.7957)
  line L582 (90.1625, -70.7957) -> (90.1948, -70.8067)
  line L583 (96.16, -71.2311) -> (96.16, -72.2788)
  line L584 (90.1074, -72.1288) -> (90.2125, -72.0587)
  line L585 (96.073, -70.9742) -> (96.0745, -70.9817)
  line L586 (90.3789, -70.9159) -> (90.4301, -70.9742)
  line L587 (96.16, -72.2788) -> (96.1399, -72.3538)
  line L588 (95.5029, -70.819) -> (95.5064, -70.8155)
  line L589 (89.9125, -71.0954) -> (89.8288, -71.1512)
  line L590 (95.2171, -70.9454) -> (95.2372, -70.8704)
  line L591 (90.4454, -71.0503) -> (90.4205, -71.1239)
  line L592 (95.5064, -70.8155) -> (95.5394, -70.8067)
  line L593 (90.286, -71.1904) -> (90.2125, -71.1655)
  line L594 (89.6243, -72.2892) -> (89.6043, -72.2735)
  line L595 (90.2278, -70.8155) -> (90.2313, -70.819)
  line L596 (90.1625, -72.4284) -> (90.1576, -72.4275)
  line L597 (89.6043, -72.2735) -> (89.5328, -72.1783)
  line L598 (89.4314, -71.8978) -> (89.4314, -71.3264)
  line L599 (90.1074, -71.0954) -> (89.9125, -71.0954)
  line L600 (89.441, -71.2737) -> (89.5124, -71.0832)
  line L601 (90.4454, -72.1739) -> (90.4301, -72.25)
  line L602 (90.4301, -72.25) -> (90.3789, -72.3083)
  line L603 (90.3622, -72.0491) -> (90.4205, -72.1003)
  line L604 (89.4384, -71.3004) -> (89.441, -71.2737)
  line L605 (90.2278, -72.4087) -> (90.1948, -72.4175)
  line L606 (90.1528, -72.4288) -> (89.8671, -72.4288)
  line L607 (89.5328, -72.1783) -> (89.5248, -72.1584)
  line L608 (89.5124, -72.141) -> (89.441, -71.9505)
  line L609 (89.7921, -72.4087) -> (89.7886, -72.4052)
  line L610 (90.1948, -72.4175) -> (90.1625, -72.4284)
  line L611 (89.8251, -72.4175) -> (89.7921, -72.4087)
  line L612 (89.5248, -72.1584) -> (89.5124, -72.141)
  line L613 (90.1576, -72.4275) -> (90.1528, -72.4288)
  line L614 (89.8623, -72.4275) -> (89.8575, -72.4284)
  line L615 (89.8671, -72.4288) -> (89.8623, -72.4275)
  line L616 (89.4384, -71.9238) -> (89.4314, -71.8978)
  line L617 (90.236, -72.4036) -> (90.2313, -72.4052)
  line L618 (89.4314, -71.3264) -> (89.4384, -71.3004)
  line L619 (89.7886, -72.4052) -> (89.7839, -72.4036)
  line L620 (89.441, -71.9505) -> (89.4384, -71.9238)
  line L621 (89.6411, -72.3083) -> (89.6243, -72.2892)
  line L622 (89.8575, -72.4284) -> (89.8251, -72.4175)
  line L623 (89.5328, -71.0459) -> (89.6043, -70.9507)
  line L624 (90.2313, -72.4052) -> (90.2278, -72.4087)
  line L625 (89.8251, -70.8067) -> (89.8575, -70.7957)
  line L626 (94.5217, -72.4036) -> (94.517, -72.4052)
  line L627 (94.5135, -72.4087) -> (94.4806, -72.4175)
  line L628 (90.4205, -72.1003) -> (90.4454, -72.1739)
  line L629 (90.286, -72.0338) -> (90.3622, -72.0491)
  line L630 (90.3789, -72.3083) -> (90.236, -72.4036)
  line L631 (89.6043, -70.9507) -> (89.6243, -70.935)
  line L632 (89.6243, -70.935) -> (89.6411, -70.9159)
  line L633 (89.7839, -70.8206) -> (89.7886, -70.819)
  line L634 (89.8623, -70.7967) -> (89.8671, -70.7954)
  line L635 (89.7886, -70.819) -> (89.7921, -70.8155)
  line L636 (89.7839, -72.4036) -> (89.6411, -72.3083)
  line L637 (89.8575, -70.7957) -> (89.8623, -70.7967)
  line L638 (94.7278, -70.8155) -> (94.7827, -70.8704)
  line L639 (94.8028, -70.9454) -> (94.8028, -72.2788)
  line L640 (94.5778, -70.8155) -> (94.6528, -70.7954)
  line L641 (94.1822, -72.4175) -> (94.1493, -72.4087)
  line L642 (93.585, -71.0753) -> (93.51, -71.0954)
  line L643 (93.0229, -72.3538) -> (93.0028, -72.2788)
  line L644 (93.585, -70.1489) -> (93.6399, -70.2038)
  line L645 (90.1528, -70.7954) -> (90.1576, -70.7967)
  line L646 (94.5778, -72.4087) -> (94.5523, -72.3832)
  line L647 (94.4482, -72.4284) -> (94.4433, -72.4275)
  line L648 (94.4433, -72.4275) -> (94.4385, -72.4288)
  line L649 (94.16, -71.9658) -> (94.2049, -72.0856)
  line L650 (94.7278, -72.4087) -> (94.6528, -72.4288)
  line L651 (93.9931, -72.3025) -> (93.9861, -72.2994)
  line L652 (93.9469, -72.25) -> (93.9454, -72.2425)
  line L653 (94.4385, -72.4288) -> (94.2243, -72.4288)
  line L654 (89.8671, -70.7954) -> (90.1528, -70.7954)
  line L655 (94.6528, -72.4288) -> (94.5778, -72.4087)
  line L656 (89.5124, -71.0832) -> (89.5248, -71.0658)
  line L657 (94.5028, -72.0383) -> (94.5028, -70.9454)
  line L658 (93.8669, -72.019) -> (93.86, -71.993)
  line L659 (94.2146, -72.4284) -> (94.1822, -72.4175)
  line L660 (94.16, -70.9454) -> (94.16, -71.9658)
  line L661 (94.6528, -70.7954) -> (94.7278, -70.8155)
  line L662 (94.1493, -72.4087) -> (94.1457, -72.4052)
  line L663 (89.7921, -70.8155) -> (89.8251, -70.8067)
  line L664 (94.01, -70.7954) -> (94.085, -70.8155)
  line L665 (94.7827, -70.8704) -> (94.8028, -70.9454)
  line L666 (93.9982, -72.3083) -> (93.9931, -72.3025)
  line L667 (93.86, -71.993) -> (93.86, -70.9454)
  line L668 (93.9454, -72.2425) -> (93.941, -72.2362)
  line L669 (93.86, -70.9454) -> (93.8801, -70.8704)
  line L670 (94.1411, -72.4036) -> (93.9982, -72.3083)
  line L671 (94.5523, -72.3832) -> (94.5217, -72.4036)
  line L672 (93.935, -70.8155) -> (94.01, -70.7954)
  line L673 (94.085, -70.8155) -> (94.1399, -70.8704)
  line L674 (94.517, -72.4052) -> (94.5135, -72.4087)
  line L675 (93.941, -72.2362) -> (93.8695, -72.0457)
  line L676 (93.8801, -70.8704) -> (93.935, -70.8155)
  line L677 (94.1457, -72.4052) -> (94.1411, -72.4036)
  line L678 (94.5028, -70.9454) -> (94.5229, -70.8704)
  line L679 (94.2049, -72.0856) -> (94.2697, -72.1288)
  line L680 (93.9861, -72.2994) -> (93.9678, -72.2737)
  line L681 (94.2195, -72.4275) -> (94.2146, -72.4284)
  line L682 (94.7827, -72.3538) -> (94.7278, -72.4087)
  line L683 (94.2697, -72.1288) -> (94.3931, -72.1288)
  line L684 (94.2243, -72.4288) -> (94.2195, -72.4275)
  line L685 (94.8028, -72.2788) -> (94.7827, -72.3538)
  line L686 (94.5229, -70.8704) -> (94.5778, -70.8155)
  line L687 (89.5248, -71.0658) -> (89.5328, -71.0459)
  line L688 (89.6411, -70.9159) -> (89.7839, -70.8206)
  line L689 (94.3931, -72.1288) -> (94.4768, -72.073)
  line L690 (93.8695, -72.0457) -> (93.8669, -72.019)
  line L691 (94.4806, -72.4175) -> (94.4482, -72.4284)
  line L692 (93.0028, -72.2788) -> (93.0028, -71.0954)
  line L693 (94.1399, -70.8704) -> (94.16, -70.9454)
  line L694 (94.4768, -72.073) -> (94.5028, -72.0383)
  line L695 (93.66, -70.2788) -> (93.6399, -70.3538)
  line L696 (93.9678, -72.2737) -> (93.9469, -72.25)
  line L697 (100.512, -72.4093) -> (100.437, -72.4288)
  line L698 (97.9421, -71.387) -> (97.997, -71.4419)
  line L699 (92.8635, -70.8155) -> (92.9385, -70.7954)
  line L700 (97.9421, -71.6468) -> (97.8671, -71.6669)
  line L701 (93.3028, -71.0954) -> (93.3028, -72.2788)
  line L702 (101.226, -72.4288) -> (101.15, -72.4093)
  line L703 (101.355, -72.3526) -> (101.3, -72.408)
  line L704 (93.1106, -70.2838) -> (93.129, -70.2582)
  line L705 (93.136, -70.255) -> (93.1411, -70.2492)
  line L706 (101.353, -71.0216) -> (101.006, -71.6121)
  line L707 (93.3671, -70.1288) -> (93.51, -70.1288)
  line L708 (93.129, -70.2582) -> (93.136, -70.255)
  line L709 (92.9385, -71.0954) -> (92.8635, -71.0753)
  line L710 (93.3028, -70.7954) -> (93.51, -70.7954)
  line L711 (93.1528, -72.4288) -> (93.0778, -72.4087)
  line L712 (100.437, -72.4288) -> (100.362, -72.408)
  line L713 (93.585, -70.8155) -> (93.6399, -70.8704)
  line L714 (101.3, -72.408) -> (101.226, -72.4288)
  line L715 (93.6399, -71.0204) -> (93.585, -71.0753)
  line L716 (93.2886, -70.1524) -> (93.2921, -70.1489)
  line L717 (93.0028, -71.0954) -> (92.9385, -71.0954)
  line L718 (92.8086, -71.0204) -> (92.7885, -70.9454)
  line L719 (93.6399, -70.8704) -> (93.66, -70.9454)
  line L720 (93.2827, -72.3538) -> (93.2278, -72.4087)
  line L721 (93.51, -71.0954) -> (93.3028, -71.0954)
  line L722 (93.51, -70.1288) -> (93.585, -70.1489)
  line L723 (93.51, -70.4288) -> (93.4125, -70.4288)
  line L724 (101.374, -72.2774) -> (101.355, -72.3526)
  line L725 (93.0898, -70.3075) -> (93.1106, -70.2838)
  line L726 (101.355, -70.8716) -> (101.374, -70.9468)
  line L727 (92.8086, -70.8704) -> (92.8635, -70.8155)
  line L728 (93.3477, -70.472) -> (93.3028, -70.5917)
  line L729 (101.006, -71.6121) -> (101.353, -72.2026)
  line L730 (93.1411, -70.2492) -> (93.2839, -70.154)
  line L731 (93.2839, -70.154) -> (93.2886, -70.1524)
  line L732 (93.3251, -70.14) -> (93.3575, -70.1291)
  line L733 (93.51, -70.7954) -> (93.585, -70.8155)
  line L734 (92.7885, -70.9454) -> (92.8086, -70.8704)
  line L735 (93.0028, -70.7954) -> (93.0028, -70.5645)
  line L736 (93.3575, -70.1291) -> (93.3623, -70.13)
  line L737 (93.3623, -70.13) -> (93.3671, -70.1288)
  line L738 (93.0028, -70.5645) -> (93.0098, -70.5385)
  line L739 (93.2921, -70.1489) -> (93.3251, -70.14)
  line L740 (93.4125, -70.4288) -> (93.3477, -70.472)
  line L741 (97.997, -71.5919) -> (97.9421, -71.6468)
  line L742 (93.3028, -70.5917) -> (93.3028, -70.7954)
  line L743 (93.0883, -70.3151) -> (93.0898, -70.3075)
  line L744 (93.6399, -70.3538) -> (93.585, -70.4087)
  line L745 (93.0778, -72.4087) -> (93.0229, -72.3538)
  line L746 (93.2278, -72.4087) -> (93.1528, -72.4288)
  line L747 (93.66, -70.9454) -> (93.6399, -71.0204)
  line L748 (101.095, -72.3549) -> (100.831, -71.9075)
  line L749 (92.8635, -71.0753) -> (92.8086, -71.0204)
  line L750 (93.585, -70.4087) -> (93.51, -70.4288)
  line L751 (93.0124, -70.5118) -> (93.0838, -70.3213)
  line L752 (101.374, -70.9468) -> (101.353, -71.0216)
  line L753 (92.9385, -70.7954) -> (93.0028, -70.7954)
  line L754 (101.353, -72.2026) -> (101.374, -72.2774)
  line L755 (93.6399, -70.2038) -> (93.66, -70.2788)
  line L756 (101.15, -72.4093) -> (101.095, -72.3549)
  line L757 (93.0098, -70.5385) -> (93.0124, -70.5118)
  line L758 (101.3, -70.8162) -> (101.355, -70.8716)
  line L759 (93.3028, -72.2788) -> (93.2827, -72.3538)
  line L760 (93.0838, -70.3213) -> (93.0883, -70.3151)
  line L761 (100.362, -72.408) -> (100.308, -72.3526)
  line L762 (88.9763, -70.1378) -> (88.9975, -70.1408)
  line L763 (89.1589, -70.3561) -> (89.1563, -70.374)
  line L764 (88.7292, -70.4329) -> (88.7261, -70.4118)
  line L765 (88.7208, -70.374) -> (88.7182, -70.3561)
  line L766 (88.8185, -70.5592) -> (88.7471, -70.464)
  line L767 (100.289, -72.2774) -> (100.309, -72.2026)
  line L768 (98.0171, -71.5169) -> (97.997, -71.5919)
  line L769 (96.5743, -71.5169) -> (96.5944, -71.4419)
  line L770 (100.831, -71.9075) -> (100.568, -72.3549)
  line L771 (100.308, -70.8716) -> (100.362, -70.8162)
  line L772 (97.8671, -71.3669) -> (97.9421, -71.387)
  line L773 (89.1509, -70.3362) -> (89.1589, -70.3561)
  line L774 (89.1479, -70.3151) -> (89.1509, -70.3362)
  line L775 (88.7261, -70.4118) -> (88.7182, -70.3919)
  line L776 (97.997, -71.4419) -> (98.0171, -71.5169)
  line L777 (96.7243, -71.6669) -> (96.6493, -71.6468)
  line L778 (100.309, -71.0216) -> (100.289, -70.9468)
  line L779 (101.226, -70.7954) -> (101.3, -70.8162)
  line L780 (89.13, -70.464) -> (89.0585, -70.5592)
  line L781 (89.0285, -70.5892) -> (89.02, -70.5927)
  line L782 (89.0285, -70.1588) -> (89.0417, -70.1756)
  line L783 (96.5944, -71.5919) -> (96.5743, -71.5169)
  line L784 (89.1367, -70.3008) -> (89.1479, -70.3151)
  line L785 (100.568, -70.8693) -> (100.831, -71.3166)
  line L786 (89.0135, -70.5991) -> (89.0047, -70.6015)
  line L787 (100.657, -71.6121) -> (100.309, -71.0216)
  line L788 (88.9565, -70.6182) -> (88.9474, -70.6169)
  line L789 (88.9565, -70.1298) -> (88.9763, -70.1378)
  line L790 (89.0417, -70.5724) -> (89.0285, -70.5892)
  line L791 (89.1589, -70.3919) -> (89.1509, -70.4118)
  line L792 (89.13, -70.284) -> (89.1367, -70.3008)
  line L793 (96.6493, -71.387) -> (96.7243, -71.3669)
  line L794 (100.568, -72.3549) -> (100.512, -72.4093)
  line L795 (97.8671, -71.6669) -> (96.7243, -71.6669)
  line L796 (100.831, -71.3166) -> (101.095, -70.8693)
  line L797 (100.309, -72.2026) -> (100.657, -71.6121)
  line L798 (89.0135, -70.1489) -> (89.02, -70.1553)
  line L799 (100.289, -70.9468) -> (100.308, -70.8716)
  line L800 (89.1563, -70.374) -> (89.1589, -70.3919)
  line L801 (100.362, -70.8162) -> (100.437, -70.7954)
  line L802 (89.02, -70.1553) -> (89.0285, -70.1588)
  line L803 (89.1509, -70.4118) -> (89.1479, -70.4329)
  line L804 (88.9474, -70.1311) -> (88.9565, -70.1298)
  line L805 (100.437, -70.7954) -> (100.512, -70.8149)
  line L806 (96.5944, -71.4419) -> (96.6493, -71.387)
  line L807 (100.308, -72.3526) -> (100.289, -72.2774)
  line L808 (100.512, -70.8149) -> (100.568, -70.8693)
  line L809 (89.02, -70.5927) -> (89.0135, -70.5991)
  line L810 (89.0417, -70.1756) -> (89.0585, -70.1888)
  line L811 (88.9975, -70.6072) -> (88.9763, -70.6102)
  line L812 (89.1367, -70.4472) -> (89.13, -70.464)
  line L813 (89.1479, -70.4329) -> (89.1367, -70.4472)
  line L814 (101.15, -70.8149) -> (101.226, -70.7954)
  line L815 (89.0047, -70.6015) -> (88.9975, -70.6072)
  line L816 (88.9975, -70.1408) -> (89.0047, -70.1465)
  line L817 (89.0047, -70.1465) -> (89.0135, -70.1489)
  line L818 (89.0585, -70.5592) -> (89.0417, -70.5724)
  line L819 (88.7182, -70.3561) -> (88.7261, -70.3362)
  line L820 (101.095, -70.8693) -> (101.15, -70.8149)
  line L821 (96.6493, -71.6468) -> (96.5944, -71.5919)
  line L822 (89.0585, -70.1888) -> (89.13, -70.284)
  line L823 (96.7243, -71.3669) -> (97.8671, -71.3669)
  line L824 (88.9763, -70.6102) -> (88.9565, -70.6182)
  line L825 (103.091, -72.4284) -> (103.086, -72.4275)
  line L826 (110.371, -70.1489) -> (110.374, -70.152)
  line L827 (103.036, -72.1288) -> (103.12, -72.073)
  line L828 (103.296, -70.7954) -> (103.371, -70.8155)
  line L829 (110.401, -70.1792) -> (110.426, -70.2038)
  line L830 (102.578, -70.8155) -> (102.653, -70.7954)
  line L831 (102.59, -72.25) -> (102.588, -72.2425)
  line L832 (102.857, -72.4284) -> (102.825, -72.4175)
  line L833 (110.374, -70.152) -> (110.378, -70.1534)
  line L834 (103.296, -72.4288) -> (103.221, -72.4087)
  line L835 (102.783, -70.8704) -> (102.803, -70.9454)
  line L836 (110.426, -70.2038) -> (110.427, -70.208)
  line L837 (110.445, -70.283) -> (110.445, -70.2873)
  line L838 (102.51, -72.019) -> (102.503, -71.993)
  line L839 (102.636, -72.3025) -> (102.629, -72.2994)
  line L840 (103.156, -72.4087) -> (103.123, -72.4175)
  line L841 (102.825, -72.4175) -> (102.792, -72.4087)
  line L842 (103.146, -72.0383) -> (103.146, -70.9454)
  line L843 (110.437, -70.2453) -> (110.446, -70.2788)
  line L844 (102.512, -72.0457) -> (102.51, -72.019)
  line L845 (102.503, -71.993) -> (102.503, -70.9454)
  line L846 (102.503, -70.9454) -> (102.523, -70.8704)
  line L847 (110.304, -70.129) -> (110.337, -70.1399)
  line L848 (103.086, -72.4275) -> (103.081, -72.4288)
  line L849 (102.523, -70.8704) -> (102.578, -70.8155)
  line L850 (103.446, -70.9454) -> (103.446, -72.2788)
  line L851 (103.146, -70.9454) -> (103.166, -70.8704)
  line L852 (102.653, -70.7954) -> (102.728, -70.8155)
  line L853 (103.165, -72.4036) -> (103.16, -72.4052)
  line L854 (102.641, -72.3083) -> (102.636, -72.3025)
  line L855 (103.221, -72.4087) -> (103.195, -72.3832)
  line L856 (102.728, -70.8155) -> (102.783, -70.8704)
  line L857 (102.784, -72.4036) -> (102.641, -72.3083)
  line L858 (103.12, -72.073) -> (103.146, -72.0383)
  line L859 (110.337, -70.1399) -> (110.371, -70.1489)
  line L860 (102.584, -72.2362) -> (102.512, -72.0457)
  line L861 (102.629, -72.2994) -> (102.611, -72.2737)
  line L862 (110.446, -70.2788) -> (110.445, -70.283)
  line L863 (102.789, -72.4052) -> (102.784, -72.4036)
  line L864 (102.588, -72.2425) -> (102.584, -72.2362)
  line L865 (103.16, -72.4052) -> (103.156, -72.4087)
  line L866 (102.803, -71.9658) -> (102.848, -72.0856)
  line L867 (103.426, -72.3538) -> (103.371, -72.4087)
  line L868 (102.803, -70.9454) -> (102.803, -71.9658)
  line L869 (103.081, -72.4288) -> (102.867, -72.4288)
  line L870 (102.913, -72.1288) -> (103.036, -72.1288)
  line L871 (110.378, -70.1534) -> (110.401, -70.1792)
  line L872 (110.43, -70.2113) -> (110.437, -70.2453)
  line L873 (102.848, -72.0856) -> (102.913, -72.1288)
  line L874 (103.166, -70.8704) -> (103.221, -70.8155)
  line L875 (110.3, -70.1299) -> (110.304, -70.129)
  line L876 (110.426, -70.3538) -> (110.422, -70.3569)
  line L877 (103.195, -72.3832) -> (103.165, -72.4036)
  line L878 (103.123, -72.4175) -> (103.091, -72.4284)
  line L879 (102.867, -72.4288) -> (102.862, -72.4275)
  line L880 (102.862, -72.4275) -> (102.857, -72.4284)
  line L881 (103.446, -72.2788) -> (103.426, -72.3538)
  line L882 (88.2933, -72.0457) -> (88.2808, -72.0632)
  line L883 (87.7639, -70.4288) -> (87.5885, -70.4288)
  line L884 (88.13, -72.2735) -> (88.1003, -72.2968)
  line L885 (104.085, -70.8155) -> (104.139, -70.8696)
  line L886 (87.3635, -72.4087) -> (87.3086, -72.3538)
  line L887 (88.2728, -72.083) -> (88.13, -72.2735)
  line L888 (103.88, -72.3538) -> (103.86, -72.2788)
  line L889 (88.1003, -72.2968) -> (88.0709, -72.3206)
  line L890 (104.16, -71.3536) -> (104.16, -72.2788)
  line L891 (103.935, -72.4087) -> (103.88, -72.3538)
  line L892 (87.9134, -70.4952) -> (87.7639, -70.4288)
  line L893 (104.212, -70.8206) -> (104.217, -70.819)
  line L894 (104.291, -70.7967) -> (104.296, -70.7954)
  line L895 (103.86, -70.9454) -> (103.88, -70.8704)
  line L896 (104.439, -70.7954) -> (104.514, -70.8155)
  line L897 (104.589, -70.9454) -> (104.568, -71.0204)
  line L898 (104.568, -71.0204) -> (104.514, -71.0753)
  line L899 (87.3635, -70.1489) -> (87.4385, -70.1288)
  line L900 (88.0792, -70.7954) -> (88.0199, -70.6373)
  line L901 (88.0709, -72.3206) -> (87.8566, -72.4158)
  line L902 (104.254, -70.8067) -> (104.286, -70.7957)
  line L903 (104.16, -72.2788) -> (104.14, -72.3538)
  line L904 (104.514, -70.8155) -> (104.568, -70.8704)
  line L905 (87.2885, -72.2788) -> (87.2885, -70.2788)
  line L906 (103.88, -70.8704) -> (103.935, -70.8155)
  line L907 (104.568, -70.8704) -> (104.589, -70.9454)
  line L908 (104.01, -72.4288) -> (103.935, -72.4087)
  line L909 (87.7639, -72.1288) -> (87.9134, -72.0623)
  line L910 (104.341, -71.0954) -> (104.257, -71.1512)
  line L911 (103.86, -72.2788) -> (103.86, -70.9454)
  line L912 (103.935, -70.8155) -> (104.01, -70.7954)